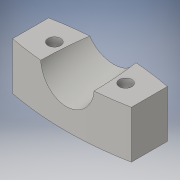
# Autodesk Inventor part: wedgeBlock
Saved by Autodesk Inventor 2016 SP1 (Build 200210100, 210)
## iProperties
Created: 2016-01-13
Part Number: wedgeBlock
Material: Generic
Document SubType Name: Modeling
Designer: ddeboer
Density: 1 g/cm^3
Appearance: Default
Author: ddeboer
Autodesk Inventor part; units mm, degrees
ref_plane "YZ Plane" through (0, 0, 0) normal (1, 0, 0) x (0, 1, 0)
ref_plane "XZ Plane" through (0, 0, 0) normal (0, 1, 0) x (-1, 0, 0)
ref_plane "XY Plane" through (0, 0, 0) normal (0, 0, 1) x (1, 0, 0)
sketch "Sketch1" plane through (0, 0, 0) normal (0, 1, 0) x (-1, 0, 0)
  line L0 (0, 0) -> (63.5, 0)
  line L1 (63.5, 0) -> (63.5, -25.4)
  line L2 (63.5, -25.4) -> (0, -25.4)
  line L3 (0, -25.4) -> (0, 0)
  dimension "d0" = 63.5
  dimension "d1" = 25.4
  constraints: 8 end point, 2 parallel, 1 horizontal, 1 perpendicular
  measures "d0" distance of L1.end L2.end
  measures "d1" distance of L2.end L0.start
extrude "Extrusion1" add sketch "Sketch1" along normal blind 25.4
sketch "Sketch2" plane through (0, 0, 0) normal (0, -1, 0) x (1, 0, 0)
  line L0 (-63.5, 0) -> (0, 0) projected
  line L1 (-31.75, 0) -> (-31.75, -25.4) construction
  line L2 (0, -25.4) -> (-63.5, -25.4) projected
  circle A0 centre (-50.8, -12.7) radius 4.7004
  circle A1 centre (-12.7, -12.7) radius 4.7004
  dimension "d4" = 19.05
  dimension "d5" = 12.7
  constraints: 2 centre point, 2 end point, 2 midpoint, 1 symmetric about line, 1 other
  measures "d4" distance from line of L1 A0.centre
  measures "d5" distance from line of A0.centre L0
hole "Hole1" at (-12.7, 0, -12.7) at (-50.8, 0, -12.7) direction (0, 1, 0) diameter 6.7564 end through all clearance for "Flat Head Machine Screw (82)" size "1/4" standard "Ansi Unified Screw Threads"
ref_plane "Work Plane1" through (0, 25.4, 0) normal (0, -0.258819, 0.9659258) x (1, 0, 0)
sketch "Sketch5" plane through (0, 25.4, 0) normal (0, -0.258819, 0.9659258) x (1, 0, 0)
  line L0 (-63.5, 0) -> (0, 0) projected
  circle A0 centre (-31.75, 0.762) radius 14.2875
  point P0 (0, -24.5345)
  dimension "d23" = 28.575
  dimension "d24" = 0.762
  constraints: 1 centre point
  measures "d23" diameter of A0
  measures "d24" distance from line of L0 A0.centre
extrude "Extrusion4" cut sketch "Sketch5" along normal mid plane 50.8
sketch "Sketch6" plane through (0, 0, 0) normal (0, -1, 0) x (1, 0, 0)
  line L0 (0, 0) -> (-63.5, 0) projected
  circle A0 centre (-31.75, -165.1) radius 165.1
  line L1 (-63.5, -25.4) -> (-63.5, 0) projected
  line L2 (-63.5, 0) -> (-63.5, -3.0816)
  line L3 (0, 0) -> (0, -3.0816)
  line L4 (0, 0) -> (0, -25.4) projected
  dimension "d28" = 330.2
  dimension "d29" = 165.1
  constraints: 4 end point, 2 point on circle, 2 point on line, 1 centre point
  measures "d28" diameter of A0
  measures "d29" distance from line of L0 A0.centre
extrude "Extrusion5" cut sketch "Sketch6" against normal blind 50.8 contours L3 A0 L0 | A0 L1 L0
sketch "Sketch7" plane through (0, 0, 0) normal (0, -1, 0) x (1, 0, 0)
  line L0 (-63.5, -25.4) -> (0, -25.4) construction
  line L1 (-31.75, -25.4) -> (-31.75, 139.7) construction
  line L2 (-31.75, -25.4) -> (133.35, -25.4) construction
  circle A0 centre (-31.75, 139.7) radius 165.1
  line L3 (0, -3.0816) -> (0, -25.4) projected
  line L4 (0, -22.3184) -> (0, -25.4)
  line L5 (0, -25.4) -> (-63.5, -25.4)
  line L6 (-63.5, -25.4) -> (-63.5, -22.3184)
  line L7 (-63.5, -25.4) -> (-63.5, -3.0816) projected
  point P0 (0, 0)
  dimension "d32" = 165.1
  dimension "d33" = 90
  constraints: 10 end point, 3 point on circle, 2 collinear, 2 point on line, 1 centre point, 1 coincident, 1 horizontal, 1 midpoint, 1 perpendicular, 1 vertical
  measures "d32" distance of L1.start L1.end
  measures "d33" angle of L2 L1
extrude "Extrusion6" cut sketch "Sketch7" against normal blind 50.8 contours A0 L5 L6 | L3 L5 A0
body "Solid1"
